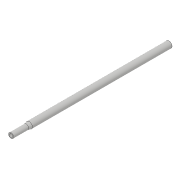
# Autodesk Inventor part: Cane Segment
Saved by Autodesk Inventor 2018.3 (Build 223284000, 284)
## iProperties
Created: 2018-11-08
Part Number: Cane Segment
Material: Generic
Document SubType Name: Modeling
Designer: aye06091
Mass: 15.2482 g
Surface Area: 228.468 cm^2
Volume: 15.2482 cm^3
Density: 1 g/cm^3
Appearance: Default
Author: aye06091
Autodesk Inventor part; units mm, degrees
ref_plane "YZ Plane" through (0, 0, 0) normal (1, 0, 0) x (0, 1, 0)
ref_plane "XZ Plane" through (0, 0, 0) normal (0, 1, 0) x (-1, 0, 0)
ref_plane "XY Plane" through (0, 0, 0) normal (0, 0, 1) x (1, 0, 0)
sketch "Sketch1" plane through (0, 0, 0) normal (0, 0, 1) x (1, 0, 0)
  circle A0 centre (0, 0) radius 6.477
  dimension "d0" = 12.954
  constraints: 1 centre point, 1 coincident
  measures "d0" diameter of A0
extrude "Extrusion1" add sketch "Sketch1" against normal blind 282.575
sketch "Sketch3" plane through (0, 0, 0) normal (0, 1, 0) x (-1, 0, 0)
  line L0 (-6.477, -282.575) -> (6.477, -282.575) projected
  line L1 (-6.477, 0) -> (6.477, 0) projected
  line L2 (6.477, 0) -> (6.477, -282.575) projected
  line L3 (-6.477, 0) -> (-6.477, -282.575) projected
  line L4 (0, 0) -> (0, 36.576)
  line L5 (5.1435, 36.576) -> (5.1435, 6.096)
  line L6 (0, 36.576) -> (5.1435, 36.576)
  line L7 (5.1435, 6.096) -> (6.477, 0)
  line L8 (6.477, 0) -> (0, 0)
  dimension "d3" = 36.576
  dimension "d4" = 5.1435
  dimension "d5" = 30.48
  constraints: 10 end point, 2 vertical, 1 collinear, 1 horizontal
  measures "d3" distance of L4.start L4.end
  measures "d4" distance between parallel lines of L4 L5
  measures "d5" distance of L5.start L5.end
revolve "Revolution1" add sketch "Sketch3" angle 360 about axis through (0, 0, 0) along (0, 0, 1) contours L1 L4 L6 L5 L7
sketch "Sketch4" plane through (0, 0, 36.576) normal (0, 0, 1) x (1, 0, 0)
  circle A0 centre (0, 0) radius 5.1435 projected
  circle A1 centre (0, 0) radius 3.6957
  dimension "d7" = 7.3914
  constraints: 1 centre point, 1 coincident
  measures "d7" diameter of A1
extrude "Extrusion2" cut sketch "Sketch4" against normal blind 36.576 contours A1
sketch "Sketch5" plane through (0, 0, -282.575) normal (0, 0, -1) x (-1, 0, 0)
  circle A0 centre (0, 0) radius 6.477 projected
  circle A1 centre (0, 0) radius 5.1562
  dimension "d10" = 10.3124
  constraints: 1 centre point, 1 coincident
  measures "d10" diameter of A1
extrude "Extrusion3" cut sketch "Sketch5" against normal blind 282.702 contours A1
body "Solid1"
